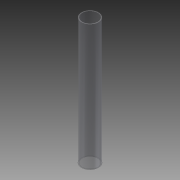
# Autodesk Inventor part: BatteryTube
Saved by Autodesk Inventor 2015 (Build 190159000, 159)
## iProperties
Created: 2014-11-25
Part Number: BatteryTube
Material: PET Plastic
Document SubType Name: Modeling
Designer: STACKPOLE
Density: 1.541 g/cm^3
Appearance: Polycarbonate - Clear
BattOD: 31.750 mm
Author: STACKPOLE
Autodesk Inventor part; units mm, degrees
ref_plane "YZ Plane" through (0, 0, 0) normal (1, 0, 0) x (0, 1, 0)
ref_plane "XZ Plane" through (0, 0, 0) normal (0, 1, 0) x (-1, 0, 0)
ref_plane "XY Plane" through (0, 0, 0) normal (0, 0, 1) x (1, 0, 0)
sketch "Sketch1" plane through (0, 0, 0) normal (0, 0, 1) x (1, 0, 0)
  circle A0 centre (0, 0) radius 15.875
  circle A1 centre (0, 0) radius 14.2875
  dimension "BattOD" = 31.75
  dimension "BattID" = 28.575
  constraints: 2 centre point, 2 coincident
  measures "BattOD" diameter of A0
  measures "BattID" diameter of A1
extrude "Extrusion1" add sketch "Sketch1" along normal blind 233
body "Solid1"
